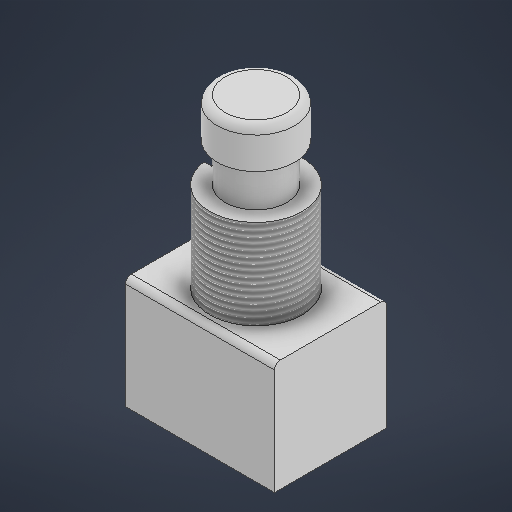
# Autodesk Inventor part: ar70736
Saved by Autodesk Inventor 2025.3 (Build 293356000, 356)
## iProperties
Created: 2026-02-28
Part Number: ar70736
Material: Generic
Document SubType Name: Modeling
Designer: Lemon
Density: 1 g/cm^3
Appearance: Default
Author: Lemon
Autodesk Inventor part; units mm, degrees
ref_plane "YZ Plane" through (0, 0, 0) normal (1, 0, 0) x (0, 1, 0)
ref_plane "XZ Plane" through (0, 0, 0) normal (0, 1, 0) x (-1, 0, 0)
ref_plane "XY Plane" through (0, 0, 0) normal (0, 0, 1) x (1, 0, 0)
sketch "Sketch1" plane through (0, 0, 0) normal (0, 1, 0) x (-1, 0, 0)
  line L0 (9.65, 7.25) -> (-9.65, 7.25)
  line L1 (-9.65, 7.25) -> (-9.65, -7.25)
  line L2 (-9.65, -7.25) -> (9.65, -7.25)
  line L3 (9.65, -7.25) -> (9.65, 7.25)
  line L4 (9.65, 7.25) -> (-9.65, -7.25) construction
  line L5 (-9.65, 7.25) -> (9.65, -7.25) construction
  point P0 (0, 0)
  dimension "d0" = 19.3
  dimension "d1" = 14.5
  constraints: 12 end point, 2 midpoint, 2 parallel, 1 horizontal, 1 perpendicular
  measures "d0" distance of L2.end L1.end
  measures "d1" distance of L1.end L0.end
extrude "Extrusion1" add sketch "Sketch1" along normal blind 14.5
sketch "Sketch2" plane through (0, 14.5, 0) normal (0, 1, 0) x (1, 0, 0)
  circle A0 centre (0, 0) radius 6
  line L0 (-6.9823, -0.8) -> (-5.0177, -0.8)
  line L1 (-5.0177, -0.8) -> (-5.0177, 0.8)
  line L2 (-5.0177, 0.8) -> (-6.9823, 0.8)
  line L3 (-6.9823, 0.8) -> (-6.9823, -0.8)
  line L4 (-6.9823, -0.8) -> (-5.0177, 0.8) construction
  line L5 (-5.0177, -0.8) -> (-6.9823, 0.8) construction
  point P0 (-6, 0)
  point P1 (5.9823, -0.4609)
  point P2 (-5.9464, -0.8)
  point P3 (-5.9464, 0.8)
  dimension "d4" = 12
  dimension "d5" = 1.6
  dimension "d6" = 11
  constraints: 12 end point, 2 midpoint, 2 parallel, 2 point on circle, 1 centre point, 1 coincident, 1 horizontal, 1 perpendicular
  measures "d4" diameter of A0
  measures "d5" distance of L0.end L1.end
  measures "d6" distance from line of A0.end L1
extrude "Extrusion2" add sketch "Sketch2" along normal blind 11.6 contours A0 L0 L1 L2 picked at (-1.3451, 0)
sketch "Sketch3" plane through (0, 26.1, 0) normal (0, 1, 0) x (1, 0, 0)
  circle A0 centre (0, 0) radius 4
  dimension "d9" = 8
  constraints: 1 centre point, 1 coincident
  measures "d9" diameter of A0
extrude "Extrusion3" add sketch "Sketch3" along normal blind 5
sketch "Sketch4" plane through (0, 31.1, 0) normal (0, 1, 0) x (1, 0, 0)
  circle A0 centre (0, 0) radius 5
  dimension "d12" = 10
  constraints: 1 centre point, 1 coincident
  measures "d12" diameter of A0
extrude "Extrusion4" add sketch "Sketch4" along normal blind 5.1
fillet "Fillet1" radius 1 1 edges at (-5, 36.2, 0)
thread "Thread1" size "M12x0.75" class "6g" standard "ANSI Metric M Profile" full length
fillet "Fillet2" radius 0.75 2 edges at (0, 14.5, 7.25) (0, 14.5, -7.25)
body "Solid1"
